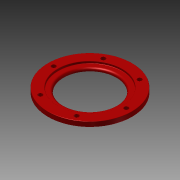
# Autodesk Inventor part: Kugel_unten_Deckel_Membran
Saved by Autodesk Inventor 2015 (Build 190159000, 159)
## iProperties
Created: 2015-07-17
Part Number: Kugel_unten_Deckel_Membran
Material: ABS-Kunststoff
Document SubType Name: Modeling
Designer: Johann
Density: 1.06 g/cm^3
Appearance: Glatt - rot
Mass: 3.20859 g
Surface Area: 33.5074 cm^2
Volume: 3.02698 cm^3
Author: Johann
Autodesk Inventor part; units mm, degrees
ref_plane "YZ Plane" through (0, 0, 0) normal (1, 0, 0) x (0, 1, 0)
ref_plane "XZ Plane" through (0, 0, 0) normal (0, 1, 0) x (-1, 0, 0)
ref_plane "XY Plane" through (0, 0, 0) normal (0, 0, 1) x (1, 0, 0)
sketch "Skizze1" plane through (0, 0, 0) normal (1, 0, 0) x (0, 1, 0)
  line L0 (0, 0) -> (0, 15)
  line L1 (18.5, 0) -> (18.5, 2)
  line L2 (18.5, 2) -> (22.5, 2)
  line L3 (22.5, 2) -> (22.5, 3.45)
  line L4 (22.5, 3.45) -> (29.5, 3.45)
  line L5 (29.5, 3.45) -> (29.5, 0)
  line L6 (29.5, 0) -> (18.5, 0)
  point P0 (24, 0)
  dimension "d0" = 15
  dimension "d1" = 45
  dimension "d2" = 7
  dimension "d3" = 37
  dimension "d24" = 2
  dimension "d25" = 1.45
  constraints: 14 end point, 5 perpendicular, 2 vertical, 1 horizontal alignment, 1 midpoint
  measures "d0" distance of L0.start L0.end
  measures "d1" diameter of L3 L0
  measures "d2" distance of L3.end L4.end
  measures "d3" diameter of L1 L0
  measures "d24" distance of L1.start L1.end
  measures "d25" distance of L2.end L3.end
revolve "Umdrehung1" add sketch "Skizze1" angle 360 about axis through (0, 0, 0) along (0, 0, 1)
sketch "Skizze2" plane through (0, 0, 0) normal (0, 0, -1) x (-1, 0, 0)
  circle A0 centre (0, 0) radius 18.5 construction
  circle A1 centre (0, 0) radius 29.5 construction
  circle A2 centre (0, 0) radius 25.5 construction
  circle A3 centre (0, 0) radius 22.5 construction
  point P0 (-25.5, 0)
  point P1 (-12.75, -22.0836)
  point P2 (12.75, -22.0836)
  point P3 (25.5, 0)
  point P4 (12.75, 22.0836)
  point P5 (-12.75, 22.0836)
  dimension "d9" = 51
  dimension "d8" = 59
  dimension "d12" = 360
  dimension "d14" = 45
  constraints: 2 horizontal alignment, 1 coincident, 9 other
  measures "d8" diameter of A1
  measures "d14" diameter of A3
hole "Bohrung1" at (25.5, 0, 0) at (12.75, -22.0836, 0) at (-12.75, -22.0836, 0) at (-25.5, 0, 0) at (-12.75, 22.0836, 0) at (12.75, 22.0836, 0) direction (0, 0, 1) diameter 3 end through all countersink diameter 4 countersink angle 90
fillet "Rundung1" radius 0.25 4 edges at (0, -22.5, 2) (0, -29.5, 3.45) (0, -29.5, 0) (0, -22.5, 3.45)
fillet "Rundung1" radius 1.5 1 edges at (0, -18.5, 2)
